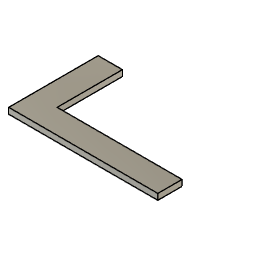
eru (Autodesk Fusion 360 design; units mm, degrees)
Autodesk Fusion 360 part; units mm, degrees
sketch "スケッチ1" plane through (0, 0, 0) normal (0, 0, 1) x (1, 0, 0)
  line L0 (0, 0) -> (250, 0)
  line L1 (250, 0) -> (250, 150)
  line L2 (250, 150) -> (0, 150)
  line L3 (0, 150) -> (0, 0)
  line L4 (250, 150) -> (40.6, 150)
  line L5 (40.6, 150) -> (40.6, 40.6)
  line L6 (40.6, 40.6) -> (250, 40.6)
  line L7 (250, 40.6) -> (250, 150)
  dimension "d1" = 250
  dimension "d2" = 150
  dimension "d3" = 40.6
  dimension "d4" = 40.6
  constraint horizontal L0
  constraint vertical L1
  constraint horizontal L2
  constraint vertical L3
  constraint coincident L0.start L3.end
  constraint horizontal L4
  constraint vertical L5
  constraint horizontal L6
  constraint vertical L7
  measures "d1" distance of L0.start L0.end
  measures "d2" distance of L0.start L2.end
  measures "d3" distance of L3 L5
  measures "d4" distance of L0 L6
extrude "押し出し1" add sketch "スケッチ1" along normal blind 10 contours L0 L1 L2 L3 L5 L6
